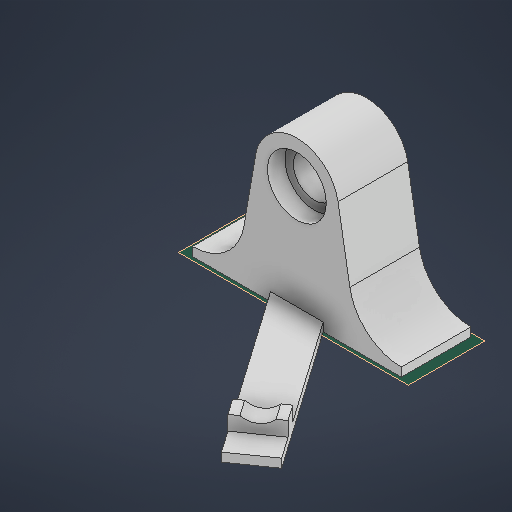
# Autodesk Inventor part: Support 2 - V1
Saved by Autodesk Inventor 2025.3 (Build 293356030, 356C)
## iProperties
Created: 2025-09-23
Part Number: Support 2 - V1
Material: Generic
Document SubType Name: Modeling
Designer: yo
Density: 1 g/cm^3
Appearance: Default
Author: yo
Autodesk Inventor part; units mm, degrees
ref_plane "YZ Plane" through (0, 0, 0) normal (1, 0, 0) x (0, 1, 0)
ref_plane "XZ Plane" through (0, 0, 0) normal (0, 1, 0) x (-1, 0, 0)
ref_plane "XY Plane" through (0, 0, 0) normal (0, 0, 1) x (1, 0, 0)
sketch "Sketch1" plane through (0, 0, 0) normal (0, 0, 1) x (1, 0, 0)
  circle A0 centre (0, 30) radius 8.45
  circle A1 centre (0, 30) radius 6
  arc A2 (-30, 0) -> (-15.2201, 12.4401) centre (-30, 15) ccw
  arc A3 (15.2201, 12.4401) -> (30, 0) centre (30, 15) ccw
  arc A4 (11.824, 32.0479) -> (-11.824, 32.0479) centre (0, 30) ccw
  line L0 (-11.824, 32.0479) -> (-15.2201, 12.4401)
  line L1 (11.824, 32.0479) -> (15.2201, 12.4401)
  line L2 (30, 0) -> (-30, 0)
  line L3 (-30, 0) -> (-30, -2.5)
  line L4 (-30, -2.5) -> (30, -2.5)
  line L5 (30, -2.5) -> (30, 0)
  point P0 (0, 0)
  point P1 (0, 0)
  point P2 (0, 0)
  dimension "d0" = 16.9
  dimension "d1" = 12
  dimension "d2" = 30
  dimension "d3" = 12
  dimension "d4" = 15
  dimension "d5" = 60
  dimension "d6" = 2.5
  constraints: 12 end point, 6 point on circle, 5 centre point, 5 tangent, 4 coincident, 2 horizontal alignment, 2 perpendicular, 2 vertical alignment, 1 equal length, 1 equal radius, 1 horizontal, 1 midpoint, 1 vertical
  measures "d0" diameter of A0
  measures "d1" diameter of A1
  measures "d2" distance of point (0, 0) A0.centre
  measures "d3" radius of A4
  measures "d4" radius of A2
  measures "d5" distance of L3.end L4.end
  measures "d6" distance of L3.start L3.end
extrude "Extrusion1" add sketch "Sketch1" along normal blind 20 contours A2 L0 A4 L1 A3 L2
extrude "Extrusion2" add sketch "Sketch1" along normal blind 15 contours A0
extrude "Extrusion3" add sketch "Sketch1" along normal blind 20 contours L2 L5 L4 L3
ref_plane "Work Plane1" through (-30, -2.5, 0) normal (0, -1, 0) x (1, 0, 0)
sketch "Sketch2" plane through (-30, -2.5, 0) normal (0, -1, 0) x (1, 0, 0)
  line L0 (21.55, 20) -> (38.45, 20) projected
  line L1 (30, 20) -> (30, 60) construction
  line L2 (60, 0) -> (60, 20) construction
  line L3 (30, 20) -> (52.9431, 52.7661) construction
  line L4 (47.9062, 63.0072) -> (64.2892, 51.5357)
  line L5 (64.2892, 51.5357) -> (61.1346, 47.0303)
  line L6 (61.1346, 47.0303) -> (44.7515, 58.5018) construction
  line L7 (44.7515, 58.5018) -> (47.9062, 63.0072)
  line L8 (44.7515, 58.5018) -> (17.7923, 20)
  line L9 (41.824, 20) -> (18.176, 20) projected
  line L10 (61.1346, 47.0303) -> (42.2077, 20)
  line L11 (0, 20) -> (60, 20) projected
  point P0 (30, 0)
  dimension "d14" = 35
  dimension "d16" = 5.5
  dimension "d17" = 20
  dimension "d26" = 40
  constraints: 16 end point, 3 parallel, 2 equal length, 2 midpoint, 2 perpendicular, 1 point on line, 1 vertical, 2 other
  measures "d14" angle of L3 L1
  measures "d16" distance of L4.end L5.end
  measures "d17" distance of L4.start L4.end
  measures "d26" distance of L1.start L1.end
extrude "Extrusion6" add sketch "Sketch2" against normal blind 2.5
sketch "Sketch4" plane through (34.2892, -2.5, 51.5357) normal (0.5735764, 0, 0.819152) x (0.819152, 0, -0.5735764)
  line L0 (-23.103, 0) -> (-34.5746, 0) projected
  circle A0 centre (-10, 10.5) radius 7.3 construction
  circle A1 centre (-10, 10.5) radius 5.35
  line L1 (-16.2022, 2.5) -> (-3.7978, 2.5)
  line L2 (-3.7978, 2.5) -> (-3.7978, 6.65)
  line L3 (-3.7978, 6.65) -> (-16.2022, 6.65)
  line L4 (-16.2022, 6.65) -> (-16.2022, 2.5)
  line L5 (-20, 2.5) -> (0, 2.5) projected
  line L6 (-16.2022, 2.5) -> (-16.2022, 0)
  line L7 (-3.7978, 2.5) -> (-3.7978, 0)
  line L8 (-23.103, 0) -> (26.0461, 0) projected
  line L9 (0, 0) -> (-20, 0) projected
  line L10 (0, 0) -> (0, 2.5) projected
  line L11 (-20, 2.5) -> (0, 2.5) projected
  line L12 (-20, 0) -> (-20, 2.5) projected
  point P0 (1.4715, 2.5)
  point P1 (-10, 2.5)
  point P2 (-6.2852, 6.65)
  point P3 (-13.7148, 6.65)
  point P4 (0, 0)
  point P5 (0, 2.5)
  point P6 (-20, 2.5)
  point P7 (-20, 0)
  point P8 (-16.2022, 2.5)
  dimension "d29" = 14.6
  dimension "d30" = 10.7
  dimension "d31" = 1.5
  dimension "d32" = 8
  constraints: 12 end point, 3 parallel, 3 point on line, 2 centre point, 2 perpendicular, 2 point on circle, 1 coincident, 1 horizontal, 1 midpoint, 1 vertical alignment
  measures "d29" diameter of A0
  measures "d30" diameter of A1
  measures "d31" distance edge to line of A1 L3
  measures "d32" distance from line of L5 A0.centre
extrude "Extrusion7" add sketch "Sketch4" against normal blind 5.5 contours A1 L3 L2 L1 L4
extrude "Extrusion8" cut sketch "Sketch4" against normal up to surface contours L6 L8 L12 L5 | L5 L10 L8 L7 surface through (0, 21, 20) normal (0, 0, 1)
extrude "Extrusion9" add sketch "Sketch4" along normal blind 7.5 contours L1 L7 L8 L6
body "Solid1"
